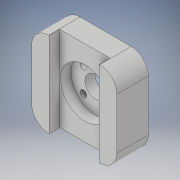
# Autodesk Inventor part: OldhamCouplerBottom
Saved by Autodesk Inventor 2018 (Build 220112000, 112)
## iProperties
Created: 2017-10-05
Part Number: OldhamCouplerBottom
Material: Generic
Document SubType Name: Modeling
Designer: Jurjen
Density: 1 g/cm^3
Appearance: Default
Author: Jurjen
Autodesk Inventor part; units mm, degrees
ref_plane "YZ Plane" through (0, 0, 0) normal (1, 0, 0) x (0, 1, 0)
ref_plane "XZ Plane" through (0, 0, 0) normal (0, 1, 0) x (-1, 0, 0)
ref_plane "XY Plane" through (0, 0, 0) normal (0, 0, 1) x (1, 0, 0)
sketch "Sketch1" plane through (0, 0, 0) normal (0, 1, 0) x (-1, 0, 0)
  line L0 (-20, 7.395) -> (-20, -7.395)
  line L1 (-20, -7.395) -> (20, -7.395)
  line L2 (20, -7.395) -> (20, 7.395)
  line L3 (20, 7.395) -> (11.74, 7.395)
  line L4 (11.74, 7.395) -> (11.74, 2.395)
  line L5 (11.74, 2.395) -> (-11.74, 2.395)
  line L6 (-11.74, 2.395) -> (-11.74, 7.395)
  line L7 (-11.74, 7.395) -> (-20, 7.395)
  point P0 (0, 0)
  point P1 (-20, 0)
  point P2 (-15.87, 7.395)
  point P3 (15.87, 7.395)
  point P4 (0, 2.395)
  dimension "d0" = 40
  dimension "d1" = 14.79
  dimension "d2" = 8.26
  dimension "d3" = 8.26
  dimension "d4" = 5
  constraints: 16 end point, 5 perpendicular, 4 midpoint, 2 horizontal alignment, 2 parallel, 1 vertical, 1 vertical alignment
  measures "d0" distance of L0.end L1.end
  measures "d1" distance of L1.end L2.end
  measures "d2" distance between parallel lines of L2 L4
  measures "d3" distance between parallel lines of L0 L6
  measures "d4" distance between parallel lines of L3 L5
extrude "Extrusion1" add sketch "Sketch1" along normal mid plane 40
sketch "Sketch2" plane through (-11.74, 20, 2.395) normal (0, 0, 1) x (1, 0, 0)
  circle A0 centre (11.74, -20) radius 11.5
  dimension "d7" = 23
  constraints: 1 centre point, 1 coincident
  measures "d7" diameter of A0
extrude "Extrusion2" cut sketch "Sketch2" against normal blind 5
sketch "Sketch3" plane through (0, 0, -2.605) normal (0, 0, 1) x (1, 0, 0)
  circle A0 centre (0, 0) radius 5
  dimension "d10" = 10
  constraints: 1 centre point, 1 coincident
  measures "d10" diameter of A0
extrude "Extrusion3" cut sketch "Sketch3" against normal up to next
sketch "Sketch4" plane through (0, 0, -2.605) normal (0, 0, 1) x (1, 0, 0)
  circle A0 centre (-5.657, 5.6575) radius 1.6
  circle A1 centre (-5.6575, -5.657) radius 1.6
  circle A2 centre (5.657, -5.6575) radius 1.6
  circle A3 centre (5.6575, 5.657) radius 1.6
  point P0 (0, 0)
  dimension "d13" = 5.657
  dimension "d14" = 5.6575
  dimension "d15" = 3.2
  dimension "d18" = 360
  constraints: 4 centre point, 9 other
  measures "d13" horizontal distance of A0.centre point (0, 0)
  measures "d14" vertical distance of point (0, 0) A0.centre
  measures "d15" diameter of A0
extrude "Extrusion4" cut sketch "Sketch4" against normal up to next
fillet "Fillet1" radius 8 4 edges at (-20, -20, 0) (20, -20, 0) (20, 20, 0) (-20, 20, 0)
body "Solid1"
